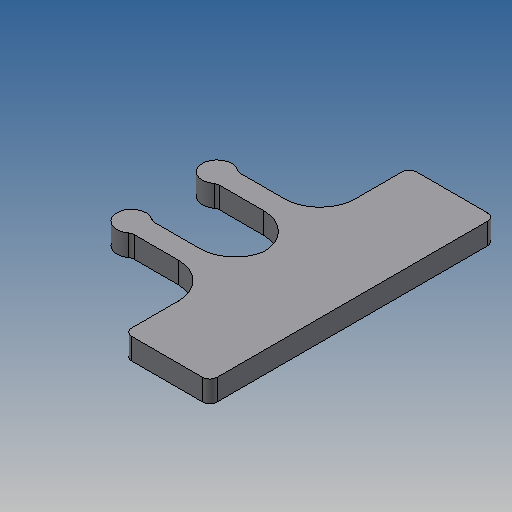
# Autodesk Inventor part: T2601_Conn
Saved by Autodesk Inventor 2025.3 (Build 293356000, 356)
## iProperties
Created: 2026-09-21
Part Number: T2601_Conn
Project: Nom Projet
Material: .
Description: Nom pièce
Document SubType Name: Modeling
Designer: jules
Authority: brut Ø
Mass: 0.00177391 g
Surface Area: 16.4276 cm^2
Volume: 1.77391 cm^3
Density: 0.001 g/cm^3
Appearance: Par défaut
Material number: ---
Author: jules
Autodesk Inventor part; units mm, degrees
ref_plane "Plan YZ" through (0, 0, 0) normal (1, 0, 0) x (0, 1, 0)
ref_plane "Plan XZ" through (0, 0, 0) normal (0, 1, 0) x (-1, 0, 0)
ref_plane "Plan XY" through (0, 0, 0) normal (0, 0, 1) x (1, 0, 0)
sketch "Esquisse1" plane through (0, 0, 0) normal (0, 0, 1) x (1, 0, 0)
  arc A0 (-11.55, 1.45) -> (-11.55, -1.45) centre (-13, 0) ccw
  line L0 (-13, 0) -> (-11.55, -1.45) construction
  line L1 (-13, 0) -> (-10.9494, 0) construction
  line L2 (-13, 0) -> (-11.55, 1.45) construction
  line L3 (-11.55, 1.45) -> (0, 1.45)
  line L4 (-11.55, -1.45) -> (0, -1.45)
  line L5 (0, -34) -> (0, 22) construction
  line L6 (-20.4607, 0) -> (17.4101, 0) construction
  line L7 (-5, -6) -> (5, -6) construction
  arc A1 (-11.55, -10.55) -> (-11.55, -13.45) centre (-13, -12) ccw
  line L8 (-11.55, -13.45) -> (0, -13.45)
  line L9 (-11.55, -10.55) -> (0, -10.55)
  line L10 (0, -26) -> (12, -26)
  line L11 (12, -26) -> (12, 14)
  line L12 (12, 14) -> (0, 14)
  line L13 (0, 14) -> (0, -26)
  line L14 (0, -26) -> (12, 14) construction
  line L15 (12, -26) -> (0, 14) construction
  point P0 (0, 0)
  point P1 (0, -6)
  point P2 (6, -6)
  point P3 (0, -13.45)
  dimension "d0" = 45
  dimension "d1" = 90
  dimension "d3" = 13
  dimension "d7" = 2.9
  dimension "d8" = 10
  dimension "d9" = 6
  dimension "d10" = 12
  dimension "d11" = 40
  constraints: 28 end point, 5 horizontal, 5 symmetric about line, 4 midpoint, 4 point on circle, 3 point on line, 2 centre point, 2 collinear, 2 parallel, 2 perpendicular, 1 equal length, 1 other
  measures "d0" angle of L0 L1
  measures "d1" angle of L0 L2
  measures "d3" distance of L0.start point (0, 0)
  measures "d7" distance between parallel lines of L4 L3
  measures "d8" distance of L7.start L7.end
  measures "d9" distance between parallel lines of L6 L7
  measures "d10" distance of L12.end L11.end
  measures "d11" distance of L11.end L10.end
extrude "Extrusion2" add sketch "Esquisse1" along normal blind 3
fillet "Congé2" radius 0.95 4 edges at (-11.55, -13.45, 1.5) (-11.55, -10.55, 1.5) (-11.55, -1.45, 1.5) (-11.55, 1.45, 1.5)
fillet "Congé3" radius 1 4 edges at (0, -26, 1.5) (12, -26, 1.5) (0, 14, 1.5) (12, 14, 1.5)
fillet "Congé4" radius 5 4 edges at (0, -13.45, 1.5) (0, -1.45, 1.5) (0, -10.55, 1.5) (0, 1.45, 1.5)
